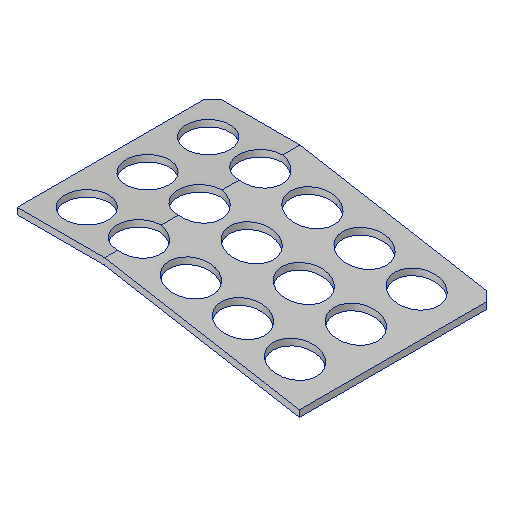
# Autodesk Inventor part: CNCM_ALU_Second_sieve
Saved by Autodesk Inventor 2025 (Build 290162010, 162A)
## iProperties
Created: 2018-09-12
Part Number: CNCM_ALU_Second_sieve
Material: Aluminum 6061
Document SubType Name: Modeling
Designer: Andrzej
Density: 2.7 g/cm^3
Appearance: Aluminum - Flat
Mass: 7.13356 g
Surface Area: 45.6681 cm^2
Volume: 2.64206 cm^3
Author: Andrzej
Autodesk Inventor part; units mm, degrees
ref_plane "YZ Plane" through (0, 0, 0) normal (1, 0, 0) x (0, 1, 0)
ref_plane "XZ Plane" through (0, 0, 0) normal (0, 1, 0) x (-1, 0, 0)
sketch "Sketch1" plane through (0, 0, 0) normal (0, 0, 1) x (1, 0, 0)
  line L0 (-25.2502, -1.5527) -> (-5.2502, -1.5527)
  line L1 (-5.2502, -1.5527) -> (39.7498, -9.4874)
  line L2 (-25.2502, -1.5527) -> (-25.2502, -0.0527)
  line L3 (-25.2502, -0.0527) -> (-5.1189, -0.0527)
  line L4 (-5.1189, -0.0527) -> (39.7498, -7.9642)
  line L5 (39.7498, -7.9642) -> (39.7498, -9.4874)
  point P0 (0, 0)
  dimension "d1" = 170
  dimension "d2" = 1.5
  dimension "d3" = 1.5
  dimension "d4" = 65
  dimension "d7" = 20
  constraints: 12 end point, 1 horizontal, 1 parallel, 1 perpendicular, 1 vertical
  measures "d1" angle of L0 L1
  measures "d2" distance of L0.start L2.end
  measures "d3" distance between parallel lines of L1 L4
  measures "d4" distance between parallel lines of L5 L2
  measures "d7" distance of L0.start L0.end
extrude "Extrusion1" add sketch "Sketch1" along normal blind 45
ref_plane "Work Plane1" through (-25.2502, -11.5527, 0) normal (0, -1, 0) x (1, 0, 0)
sketch "Sketch2" plane through (-25.2502, -11.5527, 0) normal (0, -1, 0) x (1, 0, 0)
  line L0 (20, 0) -> (65, 0) projected
  line L1 (65, 0) -> (65, 45) projected
  line L2 (20, 45) -> (65, 45) projected
  line L3 (20, 0) -> (20, 45) projected
  line L4 (0, 0) -> (20, 0) projected
  line L5 (20, 0) -> (20, 45) projected
  line L6 (0, 45) -> (20, 45) projected
  line L7 (0, 0) -> (0, 45) projected
  circle A0 centre (8, 37) radius 5
  circle A1 centre (8, 23) radius 5
  circle A2 centre (8, 9) radius 5
  circle A3 centre (20, 37) radius 5
  circle A4 centre (20, 23) radius 5
  circle A5 centre (20, 9) radius 5
  circle A6 centre (32, 37) radius 5
  circle A7 centre (32, 23) radius 5
  circle A8 centre (32, 9) radius 5
  circle A9 centre (44, 37) radius 5
  circle A10 centre (44, 23) radius 5
  circle A11 centre (44, 9) radius 5
  circle A12 centre (56, 37) radius 5
  circle A13 centre (56, 23) radius 5
  circle A14 centre (56, 9) radius 5
  point P0 (25.2502, 0)
  dimension "d9" = 10
  dimension "d10" = 8
  dimension "d11" = 8
  dimension "d14" = 14
  dimension "d17" = 12
  constraints: 15 centre point, 1 horizontal, 1 vertical, 28 other
  measures "d9" diameter of A0
  measures "d10" distance from line of L7 A0.centre
  measures "d11" distance from line of L6 A0.centre
  measures "d14" distance of A0.centre A1.centre
  measures "d17" distance of A0.centre A3.centre
extrude "Extrusion2" cut sketch "Sketch2" against normal through all contours A5 L3 | L3 A5 | A4 L3 | L3 A4 | A3 L3 | L3 A3 | A0 | A1 | A2 | A6 | A7 | A8 | A9 | A10 | A11 | A12 | A13 | A14
chamfer "Chamfer1" distance 2 angle 45 2 edges at (-25.2502, -0.8027, 0) (39.7498, -8.7258, 0)
equation "\"d3\" = d2"
equation "\"d11\" = d10"
body "Solid1"
